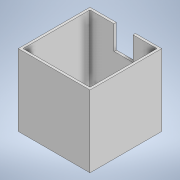
# Autodesk Inventor part: electronics bay
Saved by Autodesk Inventor 2022 (Build 260153000, 153)
## iProperties
Created: 2021-06-21
Part Number: electronics bay
Material: Generic
Document SubType Name: Modeling
Designer: WASHINGTON
Density: 1 g/cm^3
Appearance: Default
Author: WASHINGTON
Autodesk Inventor part; units mm, degrees
ref_plane "YZ Plane" through (0, 0, 0) normal (1, 0, 0) x (0, 1, 0)
ref_plane "XZ Plane" through (0, 0, 0) normal (0, 1, 0) x (-1, 0, 0)
ref_plane "XY Plane" through (0, 0, 0) normal (0, 0, 1) x (1, 0, 0)
sketch "Sketch1" plane through (0, 0, 0) normal (0, 0, 1) x (1, 0, 0)
  line L0 (0, 0) -> (-150, 0)
  line L1 (-150, 0) -> (-150, 150)
  line L2 (-150, 150) -> (0, 150)
  line L3 (0, 150) -> (0, 0)
  dimension "d0" = 150
  dimension "d1" = 150
  constraints: 8 end point, 2 parallel, 1 horizontal, 1 perpendicular
  measures "d0" distance of L0.end L1.end
  measures "d1" distance of L0.start L0.end
extrude "Extrusion1" add sketch "Sketch1" along normal mid plane 150
sketch "Sketch2" plane through (-150, 150, 75) normal (0, 1, 0) x (1, 0, 0)
  line L0 (150, 0) -> (0, 0) projected
  line L1 (150, 150) -> (150, 0) projected
  line L2 (0, 0) -> (150, 0)
  line L3 (150, 0) -> (150, 150)
  line L4 (150, 150) -> (0, 150)
  line L5 (0, 150) -> (0, 0)
  line L6 (5, 5) -> (145, 5)
  line L7 (145, 5) -> (145, 145)
  line L8 (145, 145) -> (5, 145)
  line L9 (5, 145) -> (5, 5)
  point P0 (150, 75)
  dimension "d4" = 5
  dimension "d5" = 5
  dimension "d6" = 5
  dimension "d7" = 5
  constraints: 16 end point, 4 parallel, 2 horizontal, 2 perpendicular
  measures "d4" distance between parallel lines of L5 L9
  measures "d5" distance between parallel lines of L4 L8
  measures "d6" distance between parallel lines of L0 L6
  measures "d7" distance between parallel lines of L1 L7
extrude "Extrusion2" cut sketch "Sketch2" against normal blind 145 contours L9 L8 L7 L6
sketch "Sketch3" plane through (-150, 150, 75) normal (0, 1, 0) x (1, 0, 0)
  line L0 (0, 0) -> (150, 0)
  line L1 (150, 0) -> (150, 150)
  line L2 (150, 150) -> (0, 150)
  line L3 (0, 150) -> (0, 0)
  line L4 (150, 150) -> (0, 150) projected
  line L5 (75, 150) -> (75, 0) construction
  line L6 (55, 150) -> (55, 145)
  line L7 (5, 145) -> (145, 145) construction
  line L8 (55, 145) -> (95, 145)
  line L9 (95, 150) -> (95, 145)
  point P0 (150, 75)
  dimension "d10" = 20
  dimension "d11" = 20
  constraints: 16 end point, 4 point on line, 3 parallel, 2 midpoint, 2 perpendicular, 1 horizontal
  measures "d10" distance from line of L5 L6.end
  measures "d11" distance between parallel lines of L5 L9
extrude "Extrusion3" cut sketch "Sketch3" against normal blind 50 contours L2 L9 L8 L6
body "Solid1"
